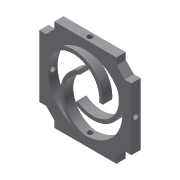
# Autodesk Inventor part: 20_Cube_Insert_Laser_Holder_v2
Saved by Autodesk Inventor 2019 (Build 230136000, 136)
## iProperties
Created: 2019-07-24
Part Number: 20_Cube_Insert_Laser_Holder_v2
Material: Generic
Document SubType Name: Modeling
Designer: marsikovabarbora
Density: 1 g/cm^3
Appearance: Default
Author: marsikovabarbora
Autodesk Inventor part; units mm, degrees
ref_plane "YZ Plane" through (0, 0, 0) normal (1, 0, 0) x (0, 1, 0)
ref_plane "XZ Plane" through (0, 0, 0) normal (0, 1, 0) x (-1, 0, 0)
ref_plane "XY Plane" through (0, 0, 0) normal (0, 0, 1) x (1, 0, 0)
sketch "Sketch1" plane through (0, 0, 0) normal (0, 0, 1) x (1, 0, 0)
  line L0 (21.5871, 13.6345) -> (17.0871, 18.1345) projected
  line L1 (17.0871, 18.1345) -> (-16.7129, 18.1345) projected
  line L2 (-16.7129, 18.1345) -> (-21.2129, 13.6345) projected
  line L3 (-21.0966, 13.6345) -> (-21.0966, -20.1655) projected
  line L4 (21.4709, -20.1655) -> (21.4709, 13.6345) projected
  line L5 (21.4709, -20.1655) -> (17.0871, -24.4078) projected
  line L6 (-16.7129, -24.4078) -> (17.0871, -24.4078) projected
  line L7 (-16.7129, -24.4078) -> (-21.0966, -20.1655) projected
  line L8 (-24.7129, -28.1655) -> (-24.7129, 13.6345) construction
  line L9 (25.0871, -28.1655) -> (-24.7129, -28.1655) construction
  line L10 (25.0871, -28.1655) -> (25.0871, 13.6345) construction
  line L11 (17.0871, 21.6345) -> (-16.7129, 21.6345) construction
  line L12 (0.1871, -36.5255) -> (0.1871, 21.9945)
  line L13 (-21.0552, -20.0655) -> (-16.6129, -24.5078)
  line L14 (-16.6129, -24.5078) -> (-16.6129, -28.1655)
  line L15 (-16.6129, -28.1655) -> (16.9871, -28.1655)
  line L16 (16.9871, -28.1655) -> (16.9871, -24.5078)
  line L17 (16.9871, -24.5078) -> (21.4295, -20.0655)
  line L18 (25.0871, -20.0655) -> (21.4295, -20.0655)
  line L19 (25.0871, 13.5345) -> (25.0871, -20.0655)
  line L20 (21.4295, 13.5345) -> (25.0871, 13.5345)
  line L21 (21.4295, 13.5345) -> (16.9871, 17.9768)
  line L22 (16.9871, 17.9768) -> (16.9871, 21.6345)
  line L23 (16.9871, 21.6345) -> (-16.6129, 21.6345)
  line L24 (-16.6129, 21.6345) -> (-16.6129, 17.9768)
  line L25 (-16.6129, 17.9768) -> (-21.0552, 13.5345)
  line L26 (-24.7129, 13.5345) -> (-21.0552, 13.5345)
  line L27 (-24.7129, -20.0655) -> (-24.7129, 13.5345)
  line L28 (-21.0552, -20.0655) -> (-24.7129, -20.0655)
  circle A0 centre (0.1871, -3.2655) radius 12.5 construction
  circle A1 centre (0.1871, -3.2655) radius 16.9 construction
  circle A2 centre (0.1871, -3.2655) radius 7.5 construction
  line L29 (0.547, -12.2476) -> (0.8041, -10.7401)
  arc A3 (-10.8411, 9.29) -> (0.8041, -10.7401) centre (-0.9086, 1.6644) ccw
  arc A4 (-14.6035, 4.5126) -> (0.547, -12.2476) centre (-0.9086, 1.6644) ccw
  arc A5 (-5.1721, -19.094) -> (6.3518, 1.0061) centre (-3.5344, -6.6794) ccw
  arc A6 (0.8464, -19.9636) -> (7.786, 1.5372) centre (-3.5344, -6.6794) ccw
  line L30 (7.786, 1.5372) -> (6.3518, 1.0061)
  arc A7 (16.5746, 0.0075) -> (-6.5945, -0.0625) centre (5.0044, -4.7815) ccw
  arc A8 (14.3185, 5.6545) -> (-7.7715, 0.914) centre (5.0044, -4.7815) ccw
  line L31 (-7.7715, 0.914) -> (-6.5945, -0.0625)
  arc A9 (0.1871, -19.9766) -> (0.8464, -19.9636) centre (0.211, -4.4767) ccw
  arc A10 (-12.8462, 5.1239) -> (-13.1888, 4.5662) centre (0.1871, -3.2655) ccw
  arc A11 (-12.8462, 5.1239) -> (-13.1888, 4.5662) centre (0.1871, -3.2655) ccw
  arc A12 (14.3185, 5.6545) -> (-10.8411, 9.29) centre (0.1871, -3.2655) ccw construction
  arc A13 (14.3185, 5.6545) -> (-10.8411, 9.29) centre (0.1871, -3.2655) ccw
  arc A14 (-14.6035, 4.5126) -> (-5.1721, -19.094) centre (0.1871, -3.2655) ccw construction
  arc A15 (0.1871, -19.9766) -> (16.5746, 0.0075) centre (0.1871, -3.2655) ccw construction
  arc A16 (-14.6035, 4.5126) -> (-5.1721, -19.094) centre (0.1871, -3.2655) ccw
  arc A17 (0.1871, -19.9766) -> (16.5746, 0.0075) centre (0.1871, -3.2655) ccw
  circle A18 centre (0.1871, -3.2655) radius 20
  point P0 (14.2, -44.8454)
  point P1 (16.9871, 19.8057)
  dimension "d49" = 15
  dimension "d48" = 25
  dimension "d53" = 360
  dimension "d61" = 40
  constraints: 40 end point, 30 point on circle, 17 centre point, 6 coincident, 6 horizontal, 6 vertical, 4 point on line, 1 midpoint, 38 other
  measures "d48" diameter of A0
  measures "d61" diameter of A18
extrude "Extrusion1" add sketch "Sketch1" along normal blind 5 contours L22 L21 L20 L4 L18 L17 L6 L12 A18 L1 | L1 L12 L23 L22 | L12 A18 L6 L13 L28 L3 L26 L25 L24 L1 | L1 L24 L23 L12 | L20 L19 L18 L4 | L12 L15 L14 L13 L6 | L6 L17 L16 L15 L12 | L3 L28 L27 L26
sketch "Sketch3" plane through (0, 0, 5) normal (0, 0, 1) x (1, 0, 0)
  circle A0 centre (0.1871, -3.2655) radius 20 projected
  circle A1 centre (0.1871, -3.2655) radius 7.5 construction
  arc A2 (-2.7759, 3.6244) -> (0.1871, -23.2655) centre (2.8116, -9.3681) ccw
  arc A3 (-3.7493, 5.3815) -> (-7.6417, -21.6695) centre (2.8116, -9.3681) ccw
  line L0 (-3.7493, 5.3815) -> (-2.7759, 3.6244)
  arc A4 (-7.6417, -21.6695) -> (0.1871, -23.2655) centre (0.1871, -3.2655) ccw
  point P0 (0, 0)
  dimension "d55" = 15
  dimension "d62" = 2
  constraints: 8 point on circle, 3 centre point, 2 coincident, 2 end point, 1 concentric, 4 other
  measures "d62" radial gap between concentric circles of A3 A2
extrude "Extrusion3" add sketch "Sketch3" against normal up to surface (5 mm away) contours A3 L0 A2 A0 picked at (-8.119, 1.4619)
pattern_circular "Circular Pattern1" count 3 over 360 about axis through (0.1871, -3.2655, 0) along (0, 0, 1) of "Extrusion3"
sketch "Sketch4" plane through (-24.7129, -20.0655, 0) normal (-1, 0, 0) x (0, 0, 1)
  line L0 (0, 41.7) -> (5, 41.7) projected
  point P0 (0, 20.0655)
  point P1 (2.5, 16.75)
  dimension "d63" = 24.95
  measures "d63" distance from line of point (2.5, 16.75) L0
hole "Hole1" at (-24.7129, -3.3155, 2.5) direction (1, 0, 0) diameter 2.9 depth 5 tip angle 118
pattern_circular "Circular Pattern2" count 4 over 360 about axis through (0.1871, -3.2655, 0) along (0, 0, 1) of "Hole1"
body "Solid1"
